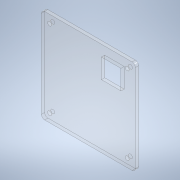
# Autodesk Inventor part: WaagePlexiTurm
Saved by Autodesk Inventor 2022 (Build 260153000, 153)
## iProperties
Created: 2021-12-03
Part Number: WaagePlexiTurm
Material: PET Plastic
Document SubType Name: Modeling
Designer: domin
Density: 1.541 g/cm^3
Appearance: Polycarbonate - Clear
Mass: 369.313 g
Surface Area: 668.72 cm^2
Volume: 239.658 cm^3
Author: domin
Autodesk Inventor part; units mm, degrees
ref_plane "YZ Plane" through (0, 0, 0) normal (1, 0, 0) x (0, 1, 0)
ref_plane "XZ Plane" through (0, 0, 0) normal (0, 1, 0) x (-1, 0, 0)
ref_plane "XY Plane" through (0, 0, 0) normal (0, 0, 1) x (1, 0, 0)
sketch "Sketch1" plane through (0, 0, 0) normal (0, 0, 1) x (1, 0, 0)
  line L0 (-72, 72) -> (72, 72)
  line L1 (72, 72) -> (72, -72)
  line L2 (72, -72) -> (-72, -72)
  line L3 (-72, -72) -> (-72, 72)
  line L4 (20, 55) -> (50, 55)
  line L5 (50, 55) -> (50, 25)
  line L6 (50, 25) -> (20, 25)
  line L7 (20, 25) -> (20, 55)
  point P0 (0, 0)
  dimension "d0" = 144
  dimension "d1" = 144
  dimension "d2" = 72
  dimension "d3" = 72
  dimension "d4" = 20
  dimension "d5" = 25
  dimension "d6" = 30
  dimension "d7" = 30
  constraints: 16 end point, 4 parallel, 2 horizontal, 2 perpendicular
  measures "d0" distance between parallel lines of L1 L3
  measures "d1" distance between parallel lines of L2 L0
  measures "d2" distance from line of point (0, 0) L3
  measures "d3" distance from line of L0 point (0, 0)
  measures "d4" distance from line of L7 point (0, 0)
  measures "d5" distance from line of point (0, 0) L6
  measures "d6" distance between parallel lines of L5 L7
  measures "d7" distance between parallel lines of L6 L4
extrude "Extrusion1" add sketch "Sketch1" along normal blind 5
fillet "Fillet1" radius 5 4 edges at (-72, -72, 2.5) (72, -72, 2.5) (72, 72, 2.5) (-72, 72, 2.5)
sketch "Sketch3" plane through (0, 0, 5) normal (0, 0, 1) x (1, 0, 0)
  line L0 (-59.5, 59.5) -> (59.5, 59.5)
  line L1 (59.5, 59.5) -> (59.5, -59.5)
  line L2 (59.5, -59.5) -> (-59.5, -59.5)
  line L3 (-59.5, -59.5) -> (-59.5, 59.5)
  circle A0 centre (-59.5, 59.5) radius 3
  point P0 (0, 0)
  dimension "d23" = 119
  dimension "d24" = 119
  dimension "d25" = 59.5
  dimension "d26" = 59.5
  dimension "d27" = 6
  constraints: 8 end point, 2 parallel, 1 centre point, 1 coincident, 1 horizontal, 1 perpendicular
  measures "d23" distance between parallel lines of L2 L0
  measures "d24" distance of L0.start L0.end
  measures "d25" distance from line of point (0, 0) L3
  measures "d26" distance from line of point (0, 0) L0
  measures "d27" diameter of A0
hole "Hole2" at (-59.5, 59.5, 5) at (59.5, 59.5, 5) at (59.5, -59.5, 5) at (-59.5, -59.5, 5) direction (0, 0, -1) diameter 6 end through all
equation "\"d2\" = 0.5 * d0"
equation "\"d3\" = 0.5 * d1"
equation "\"d25\" = 0.5 * d24"
equation "\"d26\" = 0.5 * d23"
equation "\"d28\" = d27"
body "Solid1"
